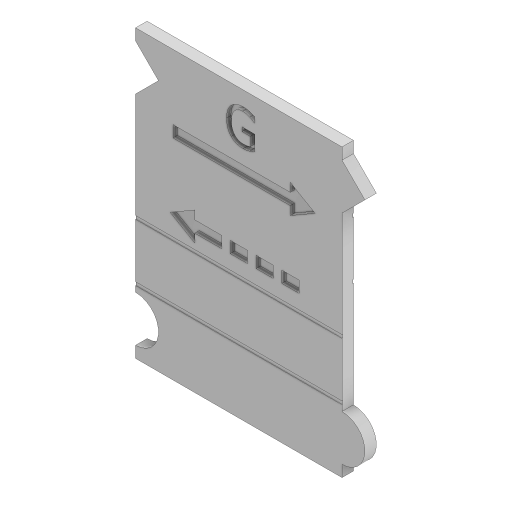
# Autodesk Inventor part: MS_G[203] text 80x60
Saved by Autodesk Inventor 2024.1 (Build 281209000, 209)
## iProperties
Created: 2023-03-29
Part Number: MS_G[203] text 80x60
Material: Generic
Document SubType Name: Modeling
Designer: LKLM8608
Density: 1 g/cm^3
Appearance: Default
Author: LKLM8608
Autodesk Inventor part; units mm, degrees
ref_plane "YZ Plane" through (0, 0, 0) normal (1, 0, 0) x (0, 1, 0)
ref_plane "XZ Plane" through (0, 0, 0) normal (0, 1, 0) x (-1, 0, 0)
sketch "Sketch1" plane through (0, 0, 0) normal (0, 0, 1) x (1, 0, 0)
  line L0 (6.0134, 0.5413) -> (-66.0587, 0.5413)
  circle A0 centre (-66.0587, 68.5413) radius 8 construction
  line L1 (-66.0587, 60.5413) -> (6.0134, 60.5413) construction
  line L2 (-66.0587, 76.5413) -> (-58.0587, 68.5413)
  line L3 (-66.0587, 60.5413) -> (-58.0587, 68.5413)
  line L4 (6.0134, 60.5413) -> (6.0134, 0.5413)
  line L5 (-66.0587, 0.5413) -> (-66.0587, 60.5413)
  line L6 (-66.0587, 76.5413) -> (-66.0587, 80.5413)
  line L7 (6.0134, 0.5413) -> (-120, 0.5413) construction
  line L8 (-60, 0) -> (-60, 75) construction
  line L9 (-60, 75) -> (0, 75) construction
  line L10 (6.0134, 150.5413) -> (6.0134, 0.5413) construction
  line L11 (6.0134, 60.5413) -> (6.0134, 80.5413)
  line L12 (-66.0587, 80.5413) -> (6.0134, 80.5413)
  line L13 (-66.0587, 76.5413) -> (12.8048, 76.5413) construction
  line L14 (-58.0587, 68.5413) -> (17.3629, 68.5413) construction
  line L15 (-66.0587, 60.5413) -> (24.3855, 60.5413) construction
  circle A1 centre (6.0134, 68.5413) radius 8 construction
  line L16 (6.0134, 60.5413) -> (14.0134, 68.5413)
  line L17 (14.0134, 68.5413) -> (6.0134, 76.5413)
  line L18 (-66.0587, 0.5413) -> (-66.0587, -7.4587) construction
  arc A2 (-66.0587, -15.4587) -> (-66.0587, 0.5413) centre (-66.0587, -7.4587) ccw
  arc A3 (6.0134, -15.4587) -> (6.0134, 0.5413) centre (6.0134, -7.4587) ccw
  line L19 (-66.0587, -15.4587) -> (-66.0587, -19.4587)
  line L20 (-66.0587, -19.4587) -> (6.0134, -19.4587)
  line L21 (6.0134, -19.4587) -> (6.0134, -15.4587)
  point P0 (0, 0)
  dimension "d1" = 80
  dimension "d5" = 16
  dimension "d6" = 60
  dimension "d132" = 8
  dimension "d133" = 4
  constraints: 44 end point, 9 point on circle, 6 perpendicular, 6 point on line, 5 horizontal, 4 centre point, 4 parallel, 4 tangent, 2 vertical, 1 coincident
  measures "d1" distance of L0.end L6.end
  measures "d5" diameter of A0
  measures "d6" distance between parallel lines of L0 L1
  measures "d132" distance of L0.end L18.end
  measures "d133" distance of L19.start L19.end
extrude "Extrusion1" add sketch "Sketch1" along normal blind 4
sketch "Sketch3" plane through (0, 0, 4) normal (0, 0, 1) x (1, 0, 0)
  line L0 (-66.0587, 80.5413) -> (13.9413, 80.5413) construction
  line L1 (-34.8487, 75.4475) -> (-28.5043, 75.4475) construction
  line L2 (-28.5043, 75.4475) -> (-28.5043, 84.7097) construction
  line L3 (-28.5043, 84.7097) -> (-34.8487, 84.7097) construction
  line L4 (-34.8487, 84.7097) -> (-34.8487, 75.4475) construction
  line L5 (-52.9694, 57.7889) -> (-12.0353, 57.7889)
  line L6 (-12.0353, 57.7889) -> (-12.0353, 60.7889)
  line L7 (-12.0353, 60.7889) -> (-3.3751, 55.7889)
  line L8 (-12.0353, 50.7889) -> (-3.3751, 55.7889)
  line L9 (-12.0353, 50.7889) -> (-12.0353, 53.7889)
  line L10 (-52.9694, 53.7889) -> (-12.0353, 53.7889)
  line L11 (-52.9694, 57.7889) -> (-52.9694, 53.7889)
  line L12 (-27, 50.7889) -> (-27, 52.7889) construction
  line L13 (-27, 35.7889) -> (-27, 32.7889) construction
  line L14 (-27, 32.7889) -> (-33, 32.7889)
  line L15 (-33, 32.7889) -> (-33, 28.7889)
  line L16 (-33, 28.7889) -> (-27, 28.7889)
  line L17 (-27, 28.7889) -> (-27, 32.7889)
  line L18 (-33, 32.7889) -> (-36, 32.7889) construction
  line L19 (-36, 32.7889) -> (-36, 28.7889)
  line L20 (-36, 32.7889) -> (-45.3694, 32.7889)
  line L21 (-45.3694, 32.7889) -> (-45.3694, 35.7889)
  line L22 (-45.3694, 35.7889) -> (-53.9694, 30.7889)
  line L23 (-36, 28.7889) -> (-45.3694, 28.7889)
  line L24 (-45.3694, 28.7889) -> (-45.3694, 25.7889)
  line L25 (-45.3694, 25.7889) -> (-53.9694, 30.7889)
  line L26 (6.0134, 0.5413) -> (-66.0587, 0.5413) construction
  line L27 (-66.0587, 80.5413) -> (6.0134, 80.5413) construction
  line L28 (-30.0226, 80.5413) -> (-30.0226, 0.5413) construction
  line L29 (-24, 32.7889) -> (-18, 32.7889)
  line L30 (-18, 32.7889) -> (-18, 28.7889)
  line L31 (-18, 28.7889) -> (-24, 28.7889)
  line L32 (-24, 28.7889) -> (-24, 32.7889)
  line L33 (-15, 32.7889) -> (-9, 32.7889)
  line L34 (-9, 32.7889) -> (-9, 28.7889)
  line L35 (-9, 28.7889) -> (-15, 28.7889)
  line L36 (-15, 28.7889) -> (-15, 32.7889)
  spline S0 degree 2 poles (-28.5015, 62.7927) (-29.7967, 62.7927) (-31.942, 63.5836) (-32.7132, 64.3844) knots 0 0 0 1 2 2 2
  spline S1 degree 2 poles (-32.7132, 64.3844) (-33.4843, 65.1951) (-34.3049, 67.5877) (-34.3049, 69.1398) knots 0 0 0 1 2 2 2
  spline S2 degree 2 poles (-34.3049, 69.1398) (-34.3049, 70.6129) (-33.4744, 72.9462) (-32.7033, 73.7766) knots 0 0 0 1 2 2 2
  spline S3 degree 2 poles (-32.7033, 73.7766) (-31.9618, 74.5774) (-29.7868, 75.4475) (-28.4916, 75.4475) knots 0 0 0 1 2 2 2
  spline S4 degree 2 poles (-28.4916, 75.4475) (-27.8688, 75.4475) (-26.7417, 75.2695) (-26.2276, 75.1113) knots 0 0 0 1 2 2 2
  spline S5 degree 2 poles (-26.2276, 75.1113) (-25.8124, 74.9927) (-24.8039, 74.5577) (-24.4975, 74.3995) knots 0 0 0 1 2 2 2
  line L37 (-24.4975, 74.3995) -> (-24.4975, 72.4419)
  line L38 (-24.4975, 72.4419) -> (-24.6359, 72.4419)
  spline S6 degree 2 poles (-24.6359, 72.4419) (-24.9424, 72.7089) (-25.585, 73.1933) (-26.1782, 73.4702) knots 0 0 0 1 2 2 2
  spline S7 degree 2 poles (-26.1782, 73.4702) (-26.6725, 73.7173) (-27.9479, 74.0436) (-28.6795, 74.0436) knots 0 0 0 1 2 2 2
  spline S8 degree 2 poles (-28.6795, 74.0436) (-30.4393, 74.0436) (-32.6143, 71.394) (-32.6143, 69.1893) knots 0 0 0 1 2 2 2
  spline S9 degree 2 poles (-32.6143, 69.1893) (-32.6143, 67.9633) (-32.0409, 66.1244) (-31.4971, 65.4917) knots 0 0 0 1 2 2 2
  spline S10 degree 2 poles (-31.4971, 65.4917) (-30.9732, 64.859) (-29.4902, 64.1966) (-28.5608, 64.1966) knots 0 0 0 1 2 2 2
  spline S11 degree 2 poles (-28.5608, 64.1966) (-27.8787, 64.1966) (-26.5143, 64.3943) (-26.0496, 64.592) knots 0 0 0 1 2 2 2
  line L39 (-26.0496, 64.592) -> (-26.0496, 67.7458)
  line L40 (-26.0496, 67.7458) -> (-28.8772, 67.7458)
  line L41 (-28.8772, 67.7458) -> (-28.8772, 69.1695)
  line L42 (-28.8772, 69.1695) -> (-24.448, 69.1695)
  line L43 (-24.448, 69.1695) -> (-24.448, 63.8407)
  spline S12 degree 2 poles (-24.448, 63.8407) (-24.7545, 63.7022) (-25.8025, 63.2771) (-26.2474, 63.1486) knots 0 0 0 1 2 2 2
  spline S13 degree 2 poles (-26.2474, 63.1486) (-26.8505, 62.9706) (-27.8193, 62.7927) (-28.5015, 62.7927) knots 0 0 0 1 2 2 2
  point P0 (-26.0587, 80.5413)
  point P1 (-12.0353, 60.7889)
  dimension "d65" = 4
  dimension "d66" = 3
  dimension "d67" = 10
  dimension "d68" = 3
  dimension "d92" = 6
  dimension "d93" = 4
  dimension "d94" = 3
  dimension "d96" = 3
  dimension "d97" = 3
  dimension "d121" = 6
  dimension "d122" = 4
  dimension "d123" = 6
  dimension "d124" = 3
  dimension "d125" = 3
  constraints: 60 end point, 6 parallel, 6 vertical, 5 horizontal, 4 perpendicular, 3 midpoint, 2 point on line, 2 other
  measures "d65" distance of L5.end L9.end
  measures "d66" distance of L5.end L6.end
  measures "d67" distance of L6.end L7.end
  measures "d68" distance of L9.end L8.start
  measures "d92" distance of L16.end L15.end
  measures "d93" distance of L15.end L14.end
  measures "d94" distance of L14.end L18.end
  measures "d96" distance of L20.end L21.end
  measures "d97" distance of L23.end L24.end
  measures "d121" distance of L30.end L31.end
  measures "d122" distance of L29.end L30.end
  measures "d123" distance of L34.end L35.end
  measures "d124" distance between parallel lines of L17 L32
  measures "d125" distance between parallel lines of L30 L36
extrude "Extrusion3" cut sketch "Sketch3" against normal blind 1.5
ref_plane "Work Plane2" through (0, 0, 0.4) normal (0, 0, -1) x (-1, 0, 0)
sketch "Sketch5" plane through (0, 0, 0.4) normal (0, 0, -1) x (-1, 0, 0)
  line L0 (-13.9413, 80.5413) -> (66.0587, 80.5413) construction
  line L1 (-6.0134, 0.5413) -> (-6.0134, 76.5413) construction
  line L2 (66.0587, 0.5413) -> (-6.0134, 0.5413) construction
  line L3 (66.0587, 60.5413) -> (66.0587, 0.5413) construction
  line L4 (66.0587, 80.5413) -> (66.0587, 76.5413) construction
  line L5 (-6.0134, 0.5413) -> (-6.0134, 60.5413) construction
  line L6 (66.0587, 60.5413) -> (66.0587, 0.5413) construction
  line L7 (58.0587, 68.5413) -> (66.0587, 60.5413) construction
  line L8 (66.0587, 76.5413) -> (58.0587, 68.5413) construction
  circle A0 centre (30.0226, 45.5413) radius 3.075
  line L9 (3.3751, 55.7889) -> (12.0353, 50.7889) construction
  line L10 (12.0353, 50.7889) -> (12.0353, 53.7889) construction
  line L11 (12.0353, 53.7889) -> (52.9694, 53.7889) construction
  line L12 (52.9694, 53.7889) -> (52.9694, 57.7889) construction
  line L13 (52.9694, 57.7889) -> (12.0353, 57.7889) construction
  line L14 (12.0353, 57.7889) -> (12.0353, 60.7889) construction
  line L15 (12.0353, 60.7889) -> (3.3751, 55.7889) construction
  line L16 (45.3694, 25.7889) -> (53.9694, 30.7889) construction
  line L17 (53.9694, 30.7889) -> (45.3694, 35.7889) construction
  line L18 (45.3694, 35.7889) -> (45.3694, 32.7889) construction
  line L19 (45.3694, 32.7889) -> (36, 32.7889) construction
  line L20 (36, 32.7889) -> (36, 28.7889) construction
  line L21 (36, 28.7889) -> (45.3694, 28.7889) construction
  line L22 (45.3694, 28.7889) -> (45.3694, 25.7889) construction
  line L23 (27, 28.7889) -> (33, 28.7889) construction
  line L24 (33, 28.7889) -> (33, 32.7889) construction
  line L25 (33, 32.7889) -> (27, 32.7889) construction
  line L26 (27, 32.7889) -> (27, 28.7889) construction
  line L27 (66.0587, 76.5413) -> (66.0587, 80.5413) construction
  line L28 (58.0587, 68.5413) -> (66.0587, 76.5413) construction
  line L29 (66.0587, 60.5413) -> (58.0587, 68.5413) construction
  line L30 (66.0587, 0.5413) -> (66.0587, 60.5413) construction
  line L31 (-6.0134, 60.5413) -> (-6.0134, 0.5413) construction
  line L32 (-6.0134, 80.5413) -> (66.0587, 80.5413) projected
  line L33 (66.0587, 80.5413) -> (-6.0134, 80.5413) projected
  line L34 (-6.0134, 76.5413) -> (-6.0134, 80.5413) projected
  line L35 (-14.0134, 68.5413) -> (-6.0134, 76.5413) projected
  line L36 (-6.0134, 60.5413) -> (-14.0134, 68.5413) projected
  line L37 (-14.0134, 68.5413) -> (-6.0134, 60.5413) projected
  line L38 (-6.0134, 76.5413) -> (-14.0134, 68.5413) projected
  line L39 (-6.0134, 80.5413) -> (-6.0134, 76.5413) projected
  arc A1 (-6.0134, 0.5413) -> (-6.0134, -15.4587) centre (-6.0134, -7.4587) ccw projected
  line L40 (-6.0134, -19.4587) -> (-6.0134, -15.4587) projected
  line L41 (66.0587, -19.4587) -> (-6.0134, -19.4587) projected
  line L42 (66.0587, -15.4587) -> (66.0587, -19.4587) projected
  arc A2 (66.0587, 0.5413) -> (66.0587, -15.4587) centre (66.0587, -7.4587) ccw projected
  arc A3 (-6.0134, 0.5413) -> (-6.0134, -15.4587) centre (-6.0134, -7.4587) ccw projected
  arc A4 (66.0587, 0.5413) -> (66.0587, -15.4587) centre (66.0587, -7.4587) ccw projected
  line L43 (66.0587, -19.4587) -> (66.0587, -15.4587) projected
  line L44 (-6.0134, -19.4587) -> (66.0587, -19.4587) projected
  line L45 (-6.0134, -15.4587) -> (-6.0134, -19.4587) projected
  dimension "d99" = 80
  dimension "d100" = 72.0721
  dimension "d101" = 6.15
  dimension "d102" = 45
  dimension "d103" = 36.036
  constraints: 1 centre point, 1 other
  measures "d99" distance between parallel lines of L0 L2
  measures "d101" diameter of A0
  measures "d102" distance from line of L2 A0.centre
  measures "d103" distance from line of L3 A0.centre
extrude "Extrusion4" cut sketch "Sketch5" against normal blind 3.15
sketch "Sketch7" plane through (0, 0, 4) normal (0, 0, 1) x (1, 0, 0)
  line L0 (-66.0587, 0.5413) -> (-66.0587, 60.5413) construction
  line L1 (6.0134, 0.5413) -> (-66.0587, 0.5413) construction
  line L2 (6.0134, 80.5413) -> (6.0134, 0.5413) construction
  line L3 (-64.0587, 23.7889) -> (4.0134, 23.7889)
  line L4 (6.0134, 2.5413) -> (-64.0587, 2.5413)
  line L5 (2.0134, 22.5889) -> (-62.0587, 22.5889)
  line L6 (-62.0587, 3.7413) -> (2.0134, 3.7413)
  line L7 (-62.0587, 22.5889) -> (-64.0587, 22.5889)
  line L8 (2.0134, 22.5889) -> (4.0134, 22.5889)
  line L9 (2.0134, 3.7413) -> (4.0134, 3.7413)
  line L10 (-62.0587, 3.7413) -> (-64.0587, 3.7413)
  line L11 (-64.0587, 23.7889) -> (-66.0587, 23.7889)
  line L12 (-64.0587, 22.5889) -> (-66.0587, 22.5889)
  line L13 (-66.0587, 23.7889) -> (-66.0587, 22.5889)
  line L14 (-64.0587, 3.7413) -> (-66.0587, 3.7413)
  line L15 (-64.0587, 2.5413) -> (-66.0587, 2.5413)
  line L16 (-66.0587, 3.7413) -> (-66.0587, 2.5413)
  line L17 (4.0134, 23.7889) -> (6.0134, 23.7889)
  line L18 (4.0134, 22.5889) -> (6.0134, 22.5889)
  line L19 (6.0134, 23.7889) -> (6.0134, 22.5889)
  line L20 (4.0134, 3.7413) -> (6.0134, 3.7413)
  line L21 (6.0134, 3.7413) -> (6.0134, 2.5413)
  point P0 (-45.3694, 25.7889)
  point P1 (6.0134, 60.5413)
  point P2 (0, 0)
  dimension "d115" = 2
  dimension "d116" = 2
  dimension "d117" = 1.2
  dimension "d120" = 1.2
  constraints: 38 end point, 10 point on line, 5 perpendicular, 4 parallel, 2 collinear, 2 horizontal, 2 vertical
  measures "d115" distance between parallel lines of L1 L4
  measures "d116" distance from line of point (-45.369, 25.789) L3
  measures "d117" distance between parallel lines of L3 L5
  measures "d120" distance between parallel lines of L4 L6
extrude "Extrusion5" cut sketch "Sketch7" against normal blind 0.2
sketch "Sketch9" plane through (0, 0, 0) normal (0, 0, -1) x (-1, 0, 0)
  line L0 (66.0587, -19.4587) -> (-6.0134, -19.4587) construction
  line L1 (-6.0134, 80.5413) -> (66.0587, 80.5413) construction
  line L2 (9, 32.7889) -> (9, 28.7889) construction
  line L3 (15, 32.7889) -> (9, 32.7889) construction
  line L4 (9, 28.7889) -> (15, 28.7889) construction
  line L5 (24.448, 69.1695) -> (24.448, 63.8407) construction
  line L6 (28.8772, 69.1695) -> (24.448, 69.1695) construction
  line L7 (28.8772, 67.7458) -> (28.8772, 69.1695) construction
  line L8 (26.0496, 67.7458) -> (28.8772, 67.7458) construction
  line L9 (26.0496, 64.592) -> (26.0496, 67.7458) construction
  line L10 (24.4975, 72.4419) -> (24.6359, 72.4419) construction
  line L11 (24.4975, 74.3995) -> (24.4975, 72.4419) construction
  line L12 (53.9694, 30.7889) -> (45.3694, 35.7889) construction
  line L13 (45.3694, 25.7889) -> (53.9694, 30.7889) construction
  line L14 (45.3694, 28.7889) -> (45.3694, 25.7889) construction
  line L15 (45.3694, 35.7889) -> (53.9694, 30.7889)
  line L16 (53.9694, 30.7889) -> (45.3694, 25.7889)
  line L17 (45.3694, 25.7889) -> (45.3694, 28.7889)
  line L18 (45.3694, 28.7889) -> (9, 28.7889)
  line L19 (9, 28.7889) -> (9, 32.7889)
  line L20 (9, 32.7889) -> (45.3694, 32.7889)
  line L21 (45.3694, 32.7889) -> (45.3694, 35.7889)
  line L22 (24.0765, 75.5669) -> (35.2096, 75.5669) construction
  line L23 (35.2096, 75.5669) -> (35.2096, 60.4551) construction
  line L24 (35.2096, 60.4551) -> (24.0765, 60.4551) construction
  line L25 (24.0765, 60.4551) -> (24.0765, 75.5669) construction
  line L26 (30.0226, 80.5413) -> (30.0226, -19.4587) construction
  line L27 (-14.0134, 68.5413) -> (58.0587, 68.5413) construction
  spline S0 degree 2 poles (30.4237, 62.9122) (29.1285, 62.9122) (26.9832, 63.7031) (26.212, 64.5039) knots 0 0 0 1 2 2 2
  spline S1 degree 2 poles (26.212, 64.5039) (25.4409, 65.3146) (24.6203, 67.7071) (24.6203, 69.2593) knots 0 0 0 1 2 2 2
  spline S2 degree 2 poles (24.6203, 69.2593) (24.6203, 70.7324) (25.4507, 73.0656) (26.2219, 73.8961) knots 0 0 0 1 2 2 2
  spline S3 degree 2 poles (26.2219, 73.8961) (26.9634, 74.6969) (29.1384, 75.5669) (30.4336, 75.5669) knots 0 0 0 1 2 2 2
  spline S4 degree 2 poles (30.4336, 75.5669) (31.0564, 75.5669) (32.1835, 75.389) (32.6976, 75.2308) knots 0 0 0 1 2 2 2
  spline S5 degree 2 poles (32.6976, 75.2308) (33.1128, 75.1122) (34.1212, 74.6772) (34.4277, 74.519) knots 0 0 0 1 2 2 2
  line L28 (34.4277, 74.519) -> (34.4277, 72.5614)
  line L29 (34.4277, 72.5614) -> (34.2893, 72.5614)
  spline S6 degree 2 poles (34.2893, 72.5614) (33.9828, 72.8284) (33.3402, 73.3128) (32.747, 73.5896) knots 0 0 0 1 2 2 2
  spline S7 degree 2 poles (32.747, 73.5896) (32.2527, 73.8368) (30.9773, 74.1631) (30.2457, 74.1631) knots 0 0 0 1 2 2 2
  spline S8 degree 2 poles (30.2457, 74.1631) (28.4859, 74.1631) (26.3109, 71.5135) (26.3109, 69.3088) knots 0 0 0 1 2 2 2
  spline S9 degree 2 poles (26.3109, 69.3088) (26.3109, 68.0828) (26.8843, 66.2439) (27.4281, 65.6112) knots 0 0 0 1 2 2 2
  spline S10 degree 2 poles (27.4281, 65.6112) (27.952, 64.9785) (29.435, 64.3161) (30.3644, 64.3161) knots 0 0 0 1 2 2 2
  spline S11 degree 2 poles (30.3644, 64.3161) (31.0465, 64.3161) (32.4109, 64.5138) (32.8755, 64.7115) knots 0 0 0 1 2 2 2
  line L30 (32.8755, 64.7115) -> (32.8755, 67.8653)
  line L31 (32.8755, 67.8653) -> (30.048, 67.8653)
  line L32 (30.048, 67.8653) -> (30.048, 69.289)
  line L33 (30.048, 69.289) -> (34.4772, 69.289)
  line L34 (34.4772, 69.289) -> (34.4772, 63.9601)
  spline S12 degree 2 poles (34.4772, 63.9601) (34.1707, 63.8217) (33.1227, 63.3966) (32.6778, 63.2681) knots 0 0 0 1 2 2 2
  spline S13 degree 2 poles (32.6778, 63.2681) (32.0747, 63.0901) (31.1058, 62.9122) (30.4237, 62.9122) knots 0 0 0 1 2 2 2
  point P0 (0, 0)
  constraints: 18 end point, 4 collinear, 3 point on line, 2 midpoint, 2 perpendicular, 16 other
extrude "Extrusion6" cut sketch "Sketch9" against normal blind 1.5
sketch "Sketch10" plane through (0, 0, 0) normal (0, 0, -1) x (-1, 0, 0)
  line L0 (-6.0134, 0.5413) -> (-6.0134, 60.5413) construction
  line L1 (66.0587, 60.5413) -> (66.0587, 0.5413) construction
  line L2 (-6.0134, 22.5889) -> (66.0587, 22.5889) construction
  line L3 (66.0587, 23.7889) -> (-6.0134, 23.7889) construction
  line L4 (66.0587, 3.7413) -> (-6.0134, 3.7413) construction
  line L5 (-6.0134, 2.5413) -> (66.0587, 2.5413) construction
  line L6 (-6.0134, 23.7889) -> (66.0587, 23.7889)
  line L7 (66.0587, 22.5889) -> (-6.0134, 22.5889)
  line L8 (-6.0134, 3.7413) -> (66.0587, 3.7413)
  line L9 (66.0587, 2.5413) -> (-6.0134, 2.5413)
  line L10 (-6.0134, 23.7889) -> (-6.0134, 22.5889)
  line L11 (66.0587, 23.7889) -> (66.0587, 22.5889)
  line L12 (66.0587, 3.7413) -> (66.0587, 2.5413)
  line L13 (-6.0134, 3.7413) -> (-6.0134, 2.5413)
  point P0 (0, 0)
  constraints: 16 end point, 7 collinear, 1 perpendicular
extrude "Extrusion7" cut sketch "Sketch10" against normal blind 0.2
sketch "Sketch11" plane through (0, 0, 0) normal (0, 0, -1) x (-1, 0, 0)
  line L0 (66.0587, 2.5413) -> (-6.0134, 2.5413) construction
  line L1 (66.0587, -19.4587) -> (-6.0134, -19.4587) construction
  arc A0 (66.0587, 0.5413) -> (66.0587, -15.4587) centre (66.0587, -7.4587) ccw construction
  line L2 (36.3941, -14.5375) -> (17.4445, -14.5375) construction
  line L3 (17.4445, -14.5375) -> (17.4445, -2.7145) construction
  line L4 (17.4445, -2.7145) -> (36.3941, -2.7145) construction
  line L5 (36.3941, -2.7145) -> (36.3941, -14.5375) construction
  line L6 (30.3756, -19.4587) -> (30.3756, 80.4905) construction
  line L7 (66.0587, -7.4587) -> (-12.2212, -7.4587) construction
  line L8 (53.9641, 30.7395) -> (53.9641, -19.4587) construction
  line L9 (9.0232, 28.6586) -> (9.0232, -19.4587) construction
  line L10 (30.3756, -1.838) -> (30.3756, 3.162) construction
  line L11 (30.3756, 3.162) -> (-6.6626, 3.162) construction
  line L12 (52.9694, 53.7889) -> (52.9694, 57.7889) construction
  line L13 (12.0353, 53.7889) -> (52.9694, 53.7889) construction
  line L14 (52.9694, 57.7889) -> (12.0353, 57.7889) construction
  line L15 (12.0353, 50.7889) -> (12.0353, 53.7889) construction
  line L16 (3.3751, 55.7889) -> (12.0353, 50.7889) construction
  line L17 (12.0353, 60.7889) -> (3.3751, 55.7889) construction
  line L18 (12.0353, 57.7889) -> (12.0353, 60.7889) construction
  line L19 (12.0716, 3.1257) -> (12.0716, 0.1257)
  line L20 (12.0716, 0.1257) -> (3.4114, 5.1257)
  line L21 (3.4114, 5.1257) -> (12.0716, 10.2095)
  line L22 (12.0716, 10.2095) -> (12.0716, 7.1257)
  line L23 (12.0716, 7.1257) -> (53.0057, 7.1257)
  line L24 (53.0057, 7.1257) -> (53.0057, 3.1257)
  line L25 (53.0057, 3.1257) -> (12.0716, 3.1257)
  spline S0 degree 2 poles (30.047, -1.8827) (31.3421, -1.8827) (33.4875, -2.6736) (34.2586, -3.4744) knots 0 0 0 1 2 2 2
  spline S1 degree 2 poles (34.2586, -3.4744) (35.0298, -4.2851) (35.8504, -6.6777) (35.8504, -8.2299) knots 0 0 0 1 2 2 2
  spline S2 degree 2 poles (35.8504, -8.2299) (35.8504, -9.703) (35.0199, -12.0362) (34.2487, -12.8667) knots 0 0 0 1 2 2 2
  spline S3 degree 2 poles (34.2487, -12.8667) (33.5073, -13.6675) (31.3322, -14.5375) (30.0371, -14.5375) knots 0 0 0 1 2 2 2
  spline S4 degree 2 poles (30.0371, -14.5375) (29.4142, -14.5375) (28.2872, -14.3595) (27.7731, -14.2013) knots 0 0 0 1 2 2 2
  spline S5 degree 2 poles (27.7731, -14.2013) (27.3578, -14.0827) (26.3494, -13.6477) (26.0429, -13.4895) knots 0 0 0 1 2 2 2
  line L26 (26.0429, -13.4895) -> (26.0429, -11.532)
  line L27 (26.0429, -11.532) -> (26.1813, -11.532)
  spline S6 degree 2 poles (26.1813, -11.532) (26.4878, -11.7989) (27.1304, -12.2834) (27.7236, -12.5602) knots 0 0 0 1 2 2 2
  spline S7 degree 2 poles (27.7236, -12.5602) (28.218, -12.8073) (29.4933, -13.1336) (30.2249, -13.1336) knots 0 0 0 1 2 2 2
  spline S8 degree 2 poles (30.2249, -13.1336) (31.9847, -13.1336) (34.1598, -10.484) (34.1598, -8.2793) knots 0 0 0 1 2 2 2
  spline S9 degree 2 poles (34.1598, -8.2793) (34.1598, -7.0534) (33.5863, -5.2145) (33.0426, -4.5817) knots 0 0 0 1 2 2 2
  spline S10 degree 2 poles (33.0426, -4.5817) (32.5186, -3.949) (31.0356, -3.2866) (30.1063, -3.2866) knots 0 0 0 1 2 2 2
  spline S11 degree 2 poles (30.1063, -3.2866) (29.4241, -3.2866) (28.0598, -3.4843) (27.5951, -3.6821) knots 0 0 0 1 2 2 2
  line L28 (27.5951, -3.6821) -> (27.5951, -6.8359)
  line L29 (27.5951, -6.8359) -> (30.4227, -6.8359)
  line L30 (30.4227, -6.8359) -> (30.4227, -8.2595)
  line L31 (30.4227, -8.2595) -> (25.9935, -8.2595)
  line L32 (25.9935, -8.2595) -> (25.9935, -2.9307)
  spline S12 degree 2 poles (25.9935, -2.9307) (26.3, -2.7923) (27.3479, -2.3671) (27.7928, -2.2386) knots 0 0 0 1 2 2 2
  spline S13 degree 2 poles (27.7928, -2.2386) (28.3959, -2.0607) (29.3648, -1.8827) (30.047, -1.8827) knots 0 0 0 1 2 2 2
  point P0 (0, 0)
  dimension "d138" = 5
  constraints: 26 end point, 7 parallel, 6 point on line, 2 perpendicular, 1 horizontal, 1 vertical, 2 other
  measures "d138" distance of L10.start L10.end
extrude "Extrusion8" cut sketch "Sketch11" against normal blind 1.5
move faces "Move3" translate (0, 0, -1.5) faces at (-33.9433, 67.0381, 1.5)
move faces "Move4" translate (0, 0, -1.5) faces at (-33.2463, 30.1222, 1.5)
move faces "Move5" translate (0, 0, -0.2) faces at (-42.0346, 22.9889, 0.2)
move faces "Move6" translate (0, 0, -0.2) faces at (-43.712, 2.7361, 0.2)
move faces "Move7" translate (0, 0, -0.2) faces at (-2.5612, 2.9413, 0.2)
sketch "Sketch12" plane through (6.0134, -19.4587, 0) normal (0, 0, -1) x (-1, 0, 0)
  line L0 (0, 20) -> (0, 80) construction
  line L1 (72.0721, 80) -> (72.0721, 20) construction
  line L2 (0, 100) -> (72.0721, 100) construction
  line L3 (72.0721, 76.8) -> (0, 76.8)
  line L4 (0, 76.8) -> (0, 78)
  line L5 (0, 78) -> (72.0721, 78)
  line L6 (72.0721, 78) -> (72.0721, 76.8)
  line L7 (72.0721, 56.752) -> (0, 56.752)
  line L8 (0, 56.752) -> (0, 57.952)
  line L9 (0, 57.952) -> (72.0721, 57.952)
  line L10 (72.0721, 57.952) -> (72.0721, 56.752)
  point P0 (6.0134, 19.4587)
  point P1 (36.036, 100)
  point P2 (36.036, 78)
  dimension "d156" = 1.2
  dimension "d157" = 22
  dimension "d158" = 1.2
  dimension "d159" = 18.848
  constraints: 16 end point, 4 parallel, 4 point on line, 2 horizontal, 2 midpoint, 2 perpendicular
  measures "d156" distance of L3.end L4.end
  measures "d157" distance of point (36.036, 100) point (36.036, 78)
  measures "d158" distance of L7.end L8.end
  measures "d159" distance between parallel lines of L9 L3
extrude "Extrusion9" cut sketch "Sketch12" against normal blind 0.2
body "Solid1"
